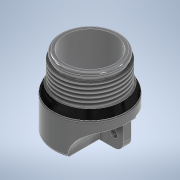
# Autodesk Inventor part: Tail Cap
Saved by Autodesk Inventor 2021 (Build 250183000, 183)
## iProperties
Created: 2020-04-08
Part Number: Tail Cap
Material: Generic
Document SubType Name: Modeling
Designer: Elijah
Density: 1 g/cm^3
Appearance: Silicon Nitride - Polished
Author: Elijah
Autodesk Inventor part; units mm, degrees
sketch "Sketch1" plane through (0, 0, 0) normal (0, 1, 0) x (-1, 0, 0)
  circle A0 centre (0, 0) radius 8.89
  dimension "d0" = 17.78
  constraints: 1 centre point, 1 coincident
  measures "d0" diameter of A0
extrude "Extrusion1" add sketch "Sketch1" along normal blind 8
sketch "Sketch2" plane through (0, 8, 0) normal (0, 1, 0) x (1, 0, 0)
  circle A0 centre (0, 0) radius 7.62
  dimension "d3" = 15.24
  constraints: 1 centre point, 1 coincident
  measures "d3" diameter of A0
extrude "Extrusion2" add sketch "Sketch2" along normal blind 0.3
ref_plane "Work Plane1" through (0, 10.3, 0) normal (0, 1, 0) x (1, 0, 0)
sketch "Sketch4" plane through (0, 10.3, 0) normal (0, 1, 0) x (1, 0, 0)
  circle A0 centre (0, 0) radius 8
  dimension "d7" = 16
  constraints: 1 centre point, 1 coincident
  measures "d7" diameter of A0
sketch "Sketch5" plane through (0, 8.3, 0) normal (0, 1, 0) x (1, 0, 0)
  circle A0 centre (0, 0) radius 8.89
  dimension "d8" = 17.78
  constraints: 1 centre point, 1 coincident
  measures "d8" diameter of A0
loft "Loft1" add profiles "Sketch5", "Sketch4"
sketch "Sketch6" plane through (0, 10.3, 0) normal (0, 1, 0) x (1, 0, 0)
  circle A0 centre (0, 0) radius 7.62
  dimension "d13" = 15.24
  constraints: 1 centre point, 1 coincident
  measures "d13" diameter of A0
extrude "Extrusion3" add sketch "Sketch6" along normal blind 5
sketch "Sketch7" plane through (0, 15.3, 0) normal (0, 1, 0) x (1, 0, 0)
  circle A0 centre (0, 0) radius 6.75
  dimension "d16" = 13.5
  constraints: 1 centre point, 1 coincident
  measures "d16" diameter of A0
ref_plane "Work Plane2" through (0, 16.3, 0) normal (0, 1, 0) x (1, 0, 0)
sketch "Sketch8" plane through (0, 16.3, 0) normal (0, 1, 0) x (1, 0, 0)
  circle A0 centre (0, 0) radius 7.25
  dimension "d18" = 14.5
  constraints: 1 centre point, 1 coincident
  measures "d18" diameter of A0
loft "Loft2" add profiles "Sketch7", "Sketch8"
fillet "Fillet1" radius 0.08 1 edges at (-8.89, 8.3, 0)
thread "Thread1" size "0.390-27 UNS" class "2A" standard "ANSI Unified Screw Threads" length 8.001
sketch "Sketch9" plane through (0, 16.3, 0) normal (0, 1, 0) x (1, 0, 0)
  circle A0 centre (0, 0) radius 7.25
  constraints: 1 centre point, 1 coincident
extrude "Extrusion4" add sketch "Sketch9" along normal blind 1
ref_plane "Work Plane3" through (0, 0, 8.89) normal (0, 0, 1) x (1, 0, 0)
sketch "Sketch10" plane through (0, 0, 8.89) normal (0, 0, 1) x (1, 0, 0)
  line L0 (8.89, 0) -> (-8.89, 0) projected
  circle A0 centre (8.89, 0) radius 5.9795
  point P0 (0, 0)
  constraints: 1 centre point
extrude "Extrusion5" cut sketch "Sketch10" against normal blind 80
ref_plane "Work Plane4" through (8.89, 0, 0) normal (1, 0, 0) x (0, 1, 0)
sketch "Sketch11" plane through (8.89, 0, 0) normal (1, 0, 0) x (0, 1, 0)
  line L0 (0, -8.89) -> (0, 8.89) projected
  line L1 (5.9795, 0.6803) -> (0, 0.6803)
  line L2 (0, 0.6803) -> (0, -1.1889)
  line L3 (0, -1.1889) -> (5.9795, -1.1889)
  line L4 (5.9795, -1.1889) -> (5.9795, 0.6803)
  point P0 (0, 0)
  point P1 (0, -8.4001)
  point P2 (0, 8.4001)
  constraints: 8 end point, 2 parallel, 1 horizontal, 1 perpendicular, 1 point on line
extrude "Extrusion6" add sketch "Sketch11" against normal up to surface
sketch "Sketch12" plane through (8.89, 0, 0.6803) normal (0, 0, 1) x (1, 0, 0)
  circle A0 centre (-2.4423, 2.9044) radius 0.889
  point P0 (-8.89, 0)
  dimension "d34" = 1.778
  constraints: 1 centre point
  measures "d34" diameter of A0
extrude "Extrusion7" cut sketch "Sketch12" against normal blind 80
fillet "Fillet2" radius 2.286 1 edges at (8.89, 0, -0.2543)
fillet "Fillet3" radius 0.5 2 edges at (-5.1555, 0, 7.2424) (-5.1555, 0, -7.2424)
fillet "Fillet4" radius 0.5 1 edges at (-7.25, 16.3, 0)
fillet "Fillet5" radius 0.5 1 edges at (-7.25, 17.3, 0)
sketch "Sketch13" plane through (0, 17.3, 0) normal (0, 1, 0) x (1, 0, 0)
  circle A0 centre (0, 0) radius 6.0809
  constraints: 1 centre point, 1 coincident
extrude "Extrusion8" cut sketch "Sketch13" against normal blind 10
body "Solid1"
